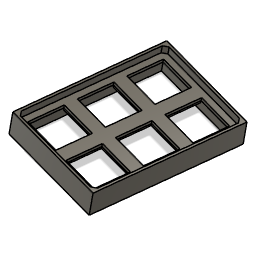
Master Assembly (Autodesk Fusion 360 archive; units mm, degrees)
design "Case Keys"
Autodesk Fusion 360 part; units mm, degrees
sketch "Sketch1" plane through (0, 0, 0) normal (0, 1, 0) x (1, 0, 0)
  line L0 (0, 0) -> (19.05, 0)
  line L1 (19.05, 0) -> (19.05, -19.05)
  line L2 (19.05, -19.05) -> (0, -19.05)
  line L3 (0, -19.05) -> (0, 0)
  line L4 (2.525, -2.525) -> (16.525, -2.525)
  line L5 (16.525, -2.525) -> (16.525, -16.525)
  line L6 (16.525, -16.525) -> (2.525, -16.525)
  line L7 (2.525, -16.525) -> (2.525, -2.525)
  line L8 (35.575, -16.525) -> (21.575, -16.525)
  line L9 (21.575, -2.525) -> (35.575, -2.525)
  line L10 (19.05, -19.05) -> (19.05, 0)
  line L11 (19.05, 0) -> (38.1, 0)
  line L12 (38.1, -19.05) -> (19.05, -19.05)
  line L13 (35.575, -2.525) -> (35.575, -16.525)
  line L14 (38.1, 0) -> (38.1, -19.05)
  line L15 (21.575, -16.525) -> (21.575, -2.525)
  line L16 (54.625, -16.525) -> (40.625, -16.525)
  line L17 (40.625, -2.525) -> (54.625, -2.525)
  line L18 (38.1, -19.05) -> (38.1, 0)
  line L19 (38.1, 0) -> (57.15, 0)
  line L20 (57.15, -19.05) -> (38.1, -19.05)
  line L21 (54.625, -2.525) -> (54.625, -16.525)
  line L22 (57.15, 0) -> (57.15, -19.05)
  line L23 (40.625, -16.525) -> (40.625, -2.525)
  line L24 (16.525, 2.525) -> (2.525, 2.525)
  line L25 (2.525, 16.525) -> (16.525, 16.525)
  line L26 (0, 0) -> (0, 19.05)
  line L27 (0, 19.05) -> (19.05, 19.05)
  line L28 (19.05, 0) -> (0, 0)
  line L29 (16.525, 16.525) -> (16.525, 2.525)
  line L30 (19.05, 19.05) -> (19.05, 0)
  line L31 (2.525, 2.525) -> (2.525, 16.525)
  line L32 (35.575, 2.525) -> (21.575, 2.525)
  line L33 (21.575, 16.525) -> (35.575, 16.525)
  line L34 (19.05, 0) -> (19.05, 19.05)
  line L35 (19.05, 19.05) -> (38.1, 19.05)
  line L36 (38.1, 0) -> (19.05, 0)
  line L37 (35.575, 16.525) -> (35.575, 2.525)
  line L38 (38.1, 19.05) -> (38.1, 0)
  line L39 (21.575, 2.525) -> (21.575, 16.525)
  line L40 (54.625, 2.525) -> (40.625, 2.525)
  line L41 (40.625, 16.525) -> (54.625, 16.525)
  line L42 (38.1, 0) -> (38.1, 19.05)
  line L43 (38.1, 19.05) -> (57.15, 19.05)
  line L44 (57.15, 0) -> (38.1, 0)
  line L45 (54.625, 16.525) -> (54.625, 2.525)
  line L46 (57.15, 19.05) -> (57.15, 0)
  line L47 (40.625, 2.525) -> (40.625, 16.525)
  line L48 (19.05, 19.05) -> (0, 19.05)
  line L49 (38.1, 19.05) -> (19.05, 19.05)
  line L50 (57.15, 19.05) -> (38.1, 19.05)
  circle A0 centre (9.525, -9.525) radius 1
  point P0 (19.05, 0)
  point P1 (38.1, 0)
  point P2 (0, 19.05)
  point P3 (19.05, 19.05)
  point P4 (38.1, 19.05)
  dimension "d13" = 19.05
  dimension "d14" = 19.05
  dimension "d15" = 2.525
  dimension "d18" = 38.1
  dimension "d19" = 38.1
  dimension "d41" = 2
  constraint horizontal L0
  constraint vertical L1
  constraint horizontal L2
  constraint vertical L3
  constraint coincident L0.start L3.end
  measures "d13" distance of L0.start L2.end
  measures "d14" distance of L0.start P0
  measures "d41" diameter of A0
extrude "Extrude1" add sketch "Sketch1" along normal blind 6.5 contours L0 L26 L27 L28 L30 L34 L48 | L0 L1 L2 L3 L10 L28 | L1 L10 L11 L12 L14 L18 L36 | L11 L30 L34 L35 L36 L38 L42 L49 | L14 L18 L19 L20 L22 L44 | L19 L38 L42 L43 L44 L46 L50
sketch "Sketch2" plane through (0, 0, 0) normal (0, 1, 0) x (1, 0, 0)
  line L0 (55.625, -17.525) -> (39.625, -17.525)
  line L1 (39.625, -17.525) -> (39.625, -1.525)
  line L2 (39.625, -1.525) -> (55.625, -1.525)
  line L3 (55.625, -1.525) -> (55.625, -17.525)
  line L4 (54.625, -16.525) -> (40.625, -16.525)
  line L5 (54.625, -2.525) -> (54.625, -16.525)
  line L6 (20.575, -1.525) -> (36.575, -1.525)
  line L7 (35.575, -2.525) -> (35.575, -16.525)
  line L8 (36.575, -1.525) -> (36.575, -17.525)
  line L9 (35.575, -16.525) -> (21.575, -16.525)
  line L10 (36.575, -17.525) -> (20.575, -17.525)
  line L11 (20.575, -17.525) -> (20.575, -1.525)
  line L12 (1.525, -1.525) -> (17.525, -1.525)
  line L13 (16.525, -2.525) -> (16.525, -16.525)
  line L14 (17.525, -1.525) -> (17.525, -17.525)
  line L15 (16.525, -16.525) -> (2.525, -16.525)
  line L16 (17.525, -17.525) -> (1.525, -17.525)
  line L17 (1.525, -17.525) -> (1.525, -1.525)
  line L18 (39.625, 17.525) -> (55.625, 17.525)
  line L19 (54.625, 16.525) -> (54.625, 2.525)
  line L20 (55.625, 17.525) -> (55.625, 1.525)
  line L21 (54.625, 2.525) -> (40.625, 2.525)
  line L22 (55.625, 1.525) -> (39.625, 1.525)
  line L23 (39.625, 1.525) -> (39.625, 17.525)
  line L24 (20.575, 17.525) -> (36.575, 17.525)
  line L25 (35.575, 16.525) -> (35.575, 2.525)
  line L26 (36.575, 17.525) -> (36.575, 1.525)
  line L27 (35.575, 2.525) -> (21.575, 2.525)
  line L28 (36.575, 1.525) -> (20.575, 1.525)
  line L29 (20.575, 1.525) -> (20.575, 17.525)
  line L30 (1.525, 17.525) -> (17.525, 17.525)
  line L31 (16.525, 16.525) -> (16.525, 2.525)
  line L32 (17.525, 17.525) -> (17.525, 1.525)
  line L33 (16.525, 2.525) -> (2.525, 2.525)
  line L34 (17.525, 1.525) -> (1.525, 1.525)
  line L35 (1.525, 1.525) -> (1.525, 17.525)
  dimension "d26" = 1
  dimension "d27" = 1
  dimension "d28" = 16
  dimension "d29" = 16
  dimension "d32" = -38.1
  dimension "d33" = 38.1
  constraint horizontal L0
  constraint vertical L1
  constraint horizontal L2
  constraint vertical L3
  measures "d26" distance of L0 L4
  measures "d27" distance of L3 L5
  measures "d28" distance of L0.start L0.end
  measures "d29" distance of L0.end L1.end
extrude "Extrude2" cut sketch "Sketch2" along normal blind 5.2
sketch "Sketch3" plane through (0, 6.5, 0) normal (0, 1, 0) x (-1, 0, 0)
  line L0 (-16.525, 16.525) -> (-2.525, 16.525)
  line L1 (-2.525, 16.525) -> (-2.525, 2.525)
  line L2 (-2.525, 2.525) -> (-16.525, 2.525)
  line L3 (-16.525, 2.525) -> (-16.525, 16.525)
  line L4 (-35.575, 16.525) -> (-21.575, 16.525)
  line L5 (-21.575, 16.525) -> (-21.575, 2.525)
  line L6 (-21.575, 2.525) -> (-35.575, 2.525)
  line L7 (-35.575, 2.525) -> (-35.575, 16.525)
  line L8 (-54.625, 16.525) -> (-40.625, 16.525)
  line L9 (-40.625, 16.525) -> (-40.625, 2.525)
  line L10 (-40.625, 2.525) -> (-54.625, 2.525)
  line L11 (-54.625, 2.525) -> (-54.625, 16.525)
  line L12 (0, -19.05) -> (0, 19.05)
  line L13 (0, 19.05) -> (-57.15, 19.05)
  line L14 (-57.15, 19.05) -> (-57.15, -19.05)
  line L15 (1, 20.05) -> (-58.15, 20.05)
  line L16 (-58.15, 20.05) -> (-58.15, -20.05)
  line L17 (-58.15, -20.05) -> (1, -20.05)
  line L18 (1, -20.05) -> (1, 20.05)
  line L19 (-57.15, -19.05) -> (0, -19.05)
  line L20 (-35.575, -2.525) -> (-21.575, -2.525)
  line L21 (-21.575, -2.525) -> (-21.575, -16.525)
  line L22 (-21.575, -16.525) -> (-35.575, -16.525)
  line L23 (-35.575, -16.525) -> (-35.575, -2.525)
  line L24 (-16.525, -2.525) -> (-2.525, -2.525)
  line L25 (-2.525, -2.525) -> (-2.525, -16.525)
  line L26 (-2.525, -16.525) -> (-16.525, -16.525)
  line L27 (-16.525, -16.525) -> (-16.525, -2.525)
  line L28 (-54.625, -2.525) -> (-40.625, -2.525)
  line L29 (-40.625, -2.525) -> (-40.625, -16.525)
  line L30 (-40.625, -16.525) -> (-54.625, -16.525)
  line L31 (-54.625, -16.525) -> (-54.625, -2.525)
  dimension "d46" = 1
  measures "d46" distance of L17 L19
extrude "Extrude3" add sketch "Sketch3" along normal blind 3 and the other way up to surface (6.5 mm away) contours L15 L16 L17 L18
sketch "Sketch4" plane through (0, 0, 0) normal (0, -1, 0) x (1, 0, 0)
  line L0 (58.15, 20.05) -> (-1, 20.05)
  line L1 (-1, 20.05) -> (-1, -20.05)
  line L2 (-1, -20.05) -> (58.15, -20.05)
  line L3 (58.15, -20.05) -> (58.15, 20.05)
  line L4 (1.525, 1.525) -> (1.525, 17.525)
  line L5 (1.525, 17.525) -> (17.525, 17.525)
  line L6 (17.525, 17.525) -> (17.525, 1.525)
  line L7 (17.525, 1.525) -> (1.525, 1.525)
  line L8 (39.625, -17.525) -> (39.625, -1.525)
  line L9 (39.625, -1.525) -> (55.625, -1.525)
  line L10 (55.625, -1.525) -> (55.625, -17.525)
  line L11 (55.625, -17.525) -> (39.625, -17.525)
  line L12 (1.525, -17.525) -> (1.525, -1.525)
  line L13 (1.525, -1.525) -> (17.525, -1.525)
  line L14 (17.525, -1.525) -> (17.525, -17.525)
  line L15 (17.525, -17.525) -> (1.525, -17.525)
  line L16 (20.575, 1.525) -> (20.575, 17.525)
  line L17 (20.575, 17.525) -> (36.575, 17.525)
  line L18 (36.575, 17.525) -> (36.575, 1.525)
  line L19 (36.575, 1.525) -> (20.575, 1.525)
  line L20 (55.625, 17.525) -> (55.625, 1.525)
  line L21 (55.625, 1.525) -> (39.625, 1.525)
  line L22 (39.625, 1.525) -> (39.625, 17.525)
  line L23 (39.625, 17.525) -> (55.625, 17.525)
  line L24 (20.575, -17.525) -> (20.575, -1.525)
  line L25 (20.575, -1.525) -> (36.575, -1.525)
  line L26 (36.575, -1.525) -> (36.575, -17.525)
  line L27 (36.575, -17.525) -> (20.575, -17.525)
  line L28 (1.525, 17.525) -> (55.625, 17.525)
  line L29 (55.625, 17.525) -> (55.625, -17.525)
  line L30 (55.625, -17.525) -> (1.525, -17.525)
  line L31 (1.525, -17.525) -> (1.525, 17.525)
  dimension "d47" = 16
  dimension "d48" = 16
  constraint horizontal L28
  constraint vertical L29
  constraint horizontal L30
  constraint vertical L31
  constraint coincident L4.end L5.start
  measures "d47" distance of L7 L4.end
  measures "d48" distance of L12.end L12.start
extrude "Extrude4" cut sketch "Sketch4" against normal blind 3 contours L4 L5 L6 L7 L28 L31 | L6 L7 L8 L9 L13 L14 L16 L18 L19 L21 L22 L24 L25 L26 L28 L29 L30 L31 | L12 L13 L14 L15 L30 L31 | L16 L17 L18 L19 L28 | L24 L25 L26 L27 L30 | L20 L21 L22 L23 L28 L29 | L8 L9 L10 L11 L29 L30
chamfer "Chamfer1" distance 1.5 angle 45 2 edges at (0, 8, 19.05) (57.15, 8, 19.05)
chamfer "Chamfer1" distance 1.5 angle 45 2 edges at (0, 8, -19.05) (57.15, 8, -19.05)
chamfer "Chamfer2" [suppressed]
chamfer "Chamfer3" [suppressed]
fillet "Fillet2" [suppressed]
chamfer "Chamfer4" [suppressed]
fillet "Fillet3" [suppressed]
